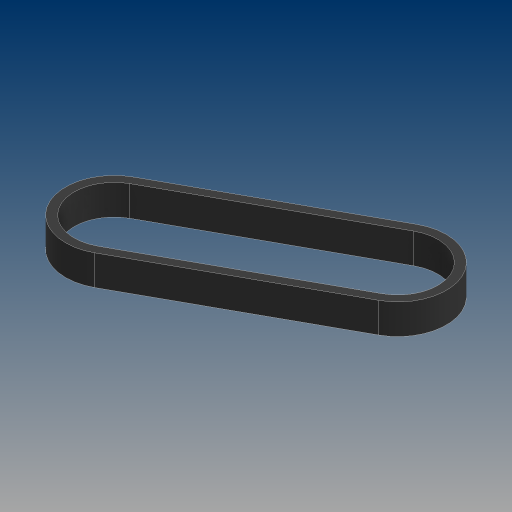
# Autodesk Inventor part: INtk_010_Belt2
Saved by Autodesk Inventor 2024.3 (Build 283343000, 343)
## iProperties
Created: 2024-08-07
Part Number: INtk_010_Belt2
Material: Rubber, Silicone
Document SubType Name: Modeling
Designer: Kenji
Density: 1.25 g/cm^3
Appearance: Rubber - Black
Author: Kenji
Autodesk Inventor part; units mm, degrees
ref_plane "YZ Plane" through (0, 0, 0) normal (1, 0, 0) x (0, 1, 0)
ref_plane "XZ Plane" through (0, 0, 0) normal (0, 1, 0) x (-1, 0, 0)
ref_plane "XY Plane" through (0, 0, 0) normal (0, 0, 1) x (1, 0, 0)
sketch "Sketch1" plane through (0, 0, 0) normal (0, 1, 0) x (-1, 0, 0)
  circle A0 centre (0, 0) radius 11.9507 construction
  line L0 (0, 0) -> (-54.7931, -30.1909) construction
  line L1 (0, 0) -> (-11.9507, 0) construction
  circle A1 centre (-54.7931, -30.1909) radius 11.9507 construction
  line L2 (-49.0258, -40.6579) -> (5.7673, -10.467)
  line L3 (-60.5604, -19.724) -> (-5.7673, 10.467)
  arc A2 (-60.5604, -19.724) -> (-49.0258, -40.6579) centre (-54.7931, -30.1909) ccw
  arc A3 (5.7673, -10.467) -> (-5.7673, 10.467) centre (0, 0) ccw
  line L4 (-6.9931, 12.6916) -> (-61.7862, -17.4993)
  arc A4 (-61.7862, -17.4993) -> (-47.8001, -42.8826) centre (-54.7931, -30.1909) ccw
  line L5 (-47.8001, -42.8826) -> (6.9931, -12.6916)
  arc A5 (6.9931, -12.6916) -> (-6.9931, 12.6916) centre (0, 0) ccw
  dimension "d11" = 23.9014
  dimension "d12" = 28.855
  dimension "d13" = 62.5602
  dimension "d14" = 2.54
  constraints: 13 point on circle, 12 end point, 7 tangent, 6 centre point, 3 coincident, 1 equal radius, 1 horizontal, 4 other
  measures "d11" diameter of A0
  measures "d12" angle of L0 L1
  measures "d13" distance of L0.start L0.end
  measures "d14" distance between parallel lines of L3 L4
extrude "Extrusion2" add sketch "Sketch1" along normal blind 8.9916
body "Solid2"
